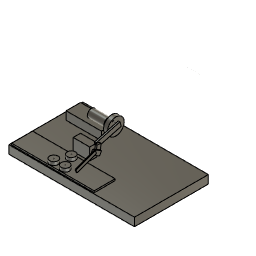
ta202 (Autodesk Fusion 360 design; units mm, degrees)
Autodesk Fusion 360 part; units mm, degrees
sketch "Sketch1" plane through (0, 0, 0) normal (0, 0, 1) x (1, 0, 0)
  line L0 (-76.1031, 44.7508) -> (76.1031, 44.7508)
  line L1 (76.1031, 44.7508) -> (76.1031, -44.7508)
  line L2 (76.1031, -44.7508) -> (-76.1031, -44.7508)
  line L3 (-76.1031, -44.7508) -> (-76.1031, 44.7508)
  line L4 (-76.1031, 44.7508) -> (76.1031, -44.7508) construction
  line L5 (76.1031, 44.7508) -> (-76.1031, -44.7508) construction
  constraint horizontal L0
  constraint perpendicular L0 L1
  constraint parallel L0 L2
  constraint parallel L1 L3
  constraint coincident L4 origin
  constraint coincident L5 origin
extrude "Extrude1" add sketch "Sketch1" along normal blind 10 makes body 1
sketch "Sketch2" plane through (0, 0, 0) normal (1, 0, 0) x (0, 1, 0)
sketch "Sketch3" plane through (0, 0, 0) normal (1, 0, 0) x (0, 1, 0)
box "BoxPrimitive1" add length 17.418 width 42.875 height 10 placed x (0, 1, 0) y (-1, 0, 0) z (0, 0, 1) at (-24.1172, 15.5422, 10) bodies 1
cylinder "CylinderPrimitive1" add diameter 10 height 20 placed x (0, 0, -1) y (0, 1, 0) z (1, 0, 0) at (0, -41.073, 85.0863) separate body makes body 2
move_face "MoveFace1" to x (1, 0, 0) y (0, 1, 0) z (0, 0, 1) at (28.6144, 17.449, -15.0737) 1 faces at (13.3333, -41.5709, 80.1111) on bodies 2
move_body "Move1" bodies 2 to x (1, 0, 0) y (0, 1, 0) z (0, 0, 1) at (-43.6789, 0, -44.4828)
sketch "Sketch6" plane through (0, 0, 0) normal (0, 1, 0) x (1, 0, 0)
move_face "MoveFace2" to x (1, 0, 0) y (0, 1, 0) z (0, 0, 1) at (0.268, 46.6265, 0) 1 faces at (-30.3455, -24.1219, 20.5547) on bodies 2
sketch "Sketch7" plane through (0, 0, 0) normal (1, 0, 0) x (0, 1, 0)
cylinder "CylinderPrimitive2" add diameter 2 height 5 placed x (0, 0, -1) y (0, 1, 0) z (1, 0, 0) at (0, -168.074, 163.9836) separate body makes body 3
move_body "Move2" bodies 3 to x (1, 0, 0) y (0, 1, 0) z (0, 0, 1) at (-21.4514, 191.469, -137.4249)
move_body "Move3" bodies 3 to x (1, 0, 0) y (0, 1, 0) z (0, 0, 1) at (-2.3482, -0.1768, -0.4425)
form "Form1" [no effect]
cylinder "CylinderPrimitive3" add diameter 20 height 5 placed x (0, 0, -1) y (0, 1, 0) z (1, 0, 0) at (0, -147.6464, 105.2635) separate body makes body 4
move_body "Move4" bodies 4 to x (1, 0, 0) y (0, 1, 0) z (0, 0, 1) at (-20, 171.5411, -79.8958)
sketch "Sketch10" plane through (0, 0, 0) normal (1, 0, 0) x (0, 1, 0)
  line L0 (-210, 70) -> (-180, 70)
  line L1 (-180, 70) -> (-180, 75.6661)
  line L2 (-180, 75.6661) -> (-210, 75.6661)
  line L3 (-210, 75.6661) -> (-210, 70)
  dimension "d14" = 30
  constraint horizontal L0
  constraint vertical L1
  constraint horizontal L2
  constraint vertical L3
  measures "d14" distance of L0.start L0.end
extrude "Extrude2" add sketch "Sketch10" along normal blind 2 separate body makes body 5
cylinder "CylinderPrimitive4" add diameter 2 height 5 placed x (0, 0, -1) y (0, 1, 0) z (1, 0, 0) at (0, -197.7484, 45.2843) separate body makes body 6
move_body "Move5" bodies 6 to x (1, 0, 0) y (0, 1, 0) z (0, 0, 1) at (-15.3609, 222.8611, -18.3783)
move_face "MoveFace3" by (0, -1.6884, -1.1256) 1 faces at (-10.3609, 25.332, 26.6123) on bodies 6
move_face "MoveFace4" to x (1, 0, 0) y (0, 1, 0) z (0, 0, 1) at (0, 0.149, -0.9888) 1 faces at (-13.6943, 25.7165, 26.1088) on bodies 6
move_body "Move6" bodies 6 to x (1, 0, 0) y (0, 1, 0) z (0, 0, 1) at (0, -2, 0)
move_body "Move7" bodies 5 to x (1, 0, 0) y (0, 1, 0) z (0, 0, 1) at (-10, 204.5024, -47.2747)
box "BoxPrimitive2" cut length 14.5484 width 8.8654 height 20 placed x (0, 0, -1) y (0, 1, 0) z (1, 0, 0) at (0, -5.9103, 24.2811) bodies 1
extrude "Extrude3" add 1 faces at (6.6667, -2.9551, 9.7327) along direction (0, 0, 1) blind 12 on bodies 1 bodies 1
move_face "MoveFace5" by (-30, 0, 3) 5 faces at (6.6667, -5.9103, 13.9109) (6.6667, -2.9551, 21.7327) (20, -2.9551, 13.9109) (6.6667, 2.9551, 13.9109) (0, -2.9551, 13.9109) on bodies 1
move_face "MoveFace6" by (0, -7, 0) 5 faces at (-10, -2.9551, 14.9109) (-23.3333, -2.9551, 24.7327) (-30, -2.9551, 14.9109) (-16.6667, 2.9551, 19.8218) (-23.3333, -5.9103, 14.9109) on bodies 1
sketch "Sketch13" plane through (0, 0, 0) normal (1, 0, 0) x (0, 1, 0)
  line L0 (-120, 50) -> (-115, 50)
  line L1 (-115, 50) -> (-115, 40)
  line L2 (-115, 40) -> (-120, 40)
  line L3 (-120, 40) -> (-120, 50)
  dimension "d26" = 5
  constraint horizontal L0
  constraint vertical L1
  constraint horizontal L2
  constraint vertical L3
  measures "d26" distance of L0.start L0.end
extrude "Extrude4" add sketch "Sketch13" along normal blind 2 separate body makes body 7
move_body "Move8" bodies 7 to x (1, 0, 0) y (0, 0.939693, -0.34202) z (0, 0.34202, 0.939693) at (-8, 89.0673, -60.0772)
sketch "Sketch14" plane through (0, 0, 0) normal (1, 0, 0) x (0, 1, 0)
  line L0 (-145, 55) -> (-140, 55)
  line L1 (-140, 55) -> (-140, 45)
  line L2 (-140, 45) -> (-145, 45)
  line L3 (-145, 45) -> (-145, 55)
  dimension "d29" = 5
  constraint horizontal L0
  constraint vertical L1
  constraint horizontal L2
  constraint vertical L3
  measures "d29" distance of L0.start L0.end
extrude "Extrude5" add sketch "Sketch14" along normal blind 2 separate body makes body 8
move_body "Move9" bodies 8 to x (1, 0, 0) y (0, 0.5, 0.866025) z (0, -0.866025, 0.5) at (7, 104.478, 118.4178)
move_body "Move10" bodies 8 to x (1, 0, 0) y (0, 1, 0) z (0, 0, 1) at (-12, 0, 0)
move_body "Move11" bodies 8 to x (1, 0, 0) y (0, 1, 0) z (0, 0, 1) at (-1, 0, 0)
sketch "Sketch15" plane through (0, 0, 0) normal (0, 0, 1) x (1, 0, 0)
  line L0 (-76.9244, -18.2082, -18.2082) -> (23.0756, -18.2082, -18.2082)
  line L1 (23.0756, -18.2082, -18.2082) -> (23.0756, -43.5769, -18.2082)
  line L2 (23.0756, -43.5769, -18.2082) -> (-76.9244, -43.5769, -18.2082)
  line L3 (-76.9244, -43.5769, -18.2082) -> (-76.9244, -18.2082, -18.2082)
  dimension "d32" = 100
extrude "Extrude6" add sketch "Sketch15" along normal blind 2 separate body contours L0 L1 L2 L3 in plane through (0, 0, -18.2082) normal (0, 0, 1) makes body 9
move_body "Move12" bodies 9 to x (1, 0, 0) y (0, 1, 0) z (0, 0, 1) at (2, 0, 30)
move_body "Move13" bodies 9 to x (1, 0, 0) y (0, 1, 0) z (0, 0, 1) at (0, 0, -1.5)
move_body "Move14" bodies 9 to x (1, 0, 0) y (0, 1, 0) z (0, 0, 1) at (1.0229, 0, -0.2046)
move_body "Move15" bodies 6 3 5 7 to x (1, 0, 0) y (0, 0.965926, 0.258819) z (0, -0.258819, 0.965926) at (0, 5.4495, 1.0154)
cylinder "CylinderPrimitive5" add diameter 10 height 4 placed x (1, 0, 0) y (0, 1, 0) z (0, 0, 1) at (-90, -90, 10) separate body makes body 10
cylinder "CylinderPrimitive6" add diameter 10 height 4 placed x (1, 0, 0) y (0, 1, 0) z (0, 0, 1) at (-72.4232, -90.9123, 10) separate body makes body 11
cylinder "CylinderPrimitive7" add diameter 10 height 4 placed x (1, 0, 0) y (0, 1, 0) z (0, 0, 1) at (-55, -90, 10) separate body makes body 12
move_body "Move16" bodies 12 to x (1, 0, 0) y (0, 1, 0) z (0, 0, 1) at (33.8754, 66.998, 2.0702)
move_body "Move17" bodies 11 to x (1, 0, 0) y (0, 1, 0) z (0, 0, 1) at (57.7763, 53.0714, 2)
move_body "Move18" bodies 10 to x (1, 0, 0) y (0, 1, 0) z (0, 0, 1) at (61.5403, 52.1304, 2)
move_face "MoveFace7" to x (1, 0, 0) y (0, 1, 0) z (0, 0, 1) at (-1, 0, 0) 2 faces at (-19.3173, -21.0864, 16.0702) (-16.1495, -23.4999, 14.7368) on bodies 12
sketch "Sketch21" plane through (0, 0, 0) normal (1, 0, 0) x (0, 1, 0)
sketch "Sketch22" plane through (0, 0, 0) normal (0, 0, 1) x (1, 0, 0)
cylinder "CylinderPrimitive8" add diameter 0.02 height 25 placed x (0, 0, -1) y (0, 1, 0) z (1, 0, 0) at (0, 91.7998, 62.8457) separate body makes body 13
cylinder "CylinderPrimitive11" add diameter 1 height 1 placed x (0, 0, -1) y (0, 1, 0) z (1, 0, 0) at (0, 68.333, 32.3551) separate body makes body 14
cylinder "CylinderPrimitive12" add diameter 1 height 1 placed x (0, 0, -1) y (0, 1, 0) z (1, 0, 0) at (0, 70, 25) separate body makes body 15
cylinder "CylinderPrimitive13" add diameter 1 height 1 placed x (0, 0, -1) y (0, 1, 0) z (1, 0, 0) at (0, 78.651, 31.8595) separate body makes body 16
cylinder "CylinderPrimitive14" add diameter 1 height 1 placed x (0, 0, -1) y (0, 1, 0) z (1, 0, 0) at (0, 78.067, 24.0747) separate body makes body 17
move_body "Move19" bodies 17 to x (1, 0, 0) y (0, 1, 0) z (0, 0, 1) at (-5.629, -57.3883, 8.9477)
move_body "Move20" bodies 15 to x (1, 0, 0) y (0, 1, 0) z (0, 0, 1) at (-1.28, -77.2263, -5.113)
move_body "Move21" bodies 14 to x (1, 0, 0) y (0, 1, 0) z (0, 0, 1) at (-1.0781, -73.9254, -5.2956)
box "BoxPrimitive4" add length 25 width 4 height 1 placed x (0, 0, 1) y (1, 0, 0) z (0, 1, 0) at (-140, 0, -79.9465) separate body makes body 18
move_body "Move23" bodies 18 to x (0, 0.173648, -0.984808) y (-1, 0, 0) z (0, 0.984808, 0.173648) at (-6.9176, 53.861, -89.1067)
move_body "Move24" bodies 18 to x (1, 0, 0) y (0, 0.984808, 0.173648) z (0, -0.173648, 0.984808) at (0, 5.6503, 6.4545)
move_body "Move25" bodies 18 to x (1, 0, 0) y (0, 1, 0) z (0, 0, 1) at (0, 12.2319, -16.2718)
move_body "Move26" bodies 14 to x (1, 0, 0) y (0, 1, 0) z (0, 0, 1) at (-5, 0, -2)
move_body "Move27" bodies 15 to x (1, 0, 0) y (0, 1, 0) z (0, 0, 1) at (-2, 0, -1)
move_body "Move28" bodies 15 to x (1, 0, 0) y (0, 1, 0) z (0, 0, 1) at (-1, 0, 0)
move_body "Move29" bodies 8 18 to x (1, 0, 0) y (0, 1, 0) z (0, 0, 1) at (20, 0, 0)
move_body "Move30" bodies 8 to x (1, 0, 0) y (0, 1, 0) z (0, 0, 1) at (-20, 0, 0)
move_body "Move31" bodies 18 to x (1, 0, 0) y (0, 1, 0) z (0, 0, 1) at (-16, 0, 0)
move_body "Move32" bodies 16 to x (1, 0, 0) y (0, 1, 0) z (0, 0, 1) at (-2.5, -92.2069, -9.2778)
move_body "Move33" bodies 16 to x (1, 0, 0) y (0, 1, 0) z (0, 0, 1) at (-0.3, 0, 0)
hole "Hole1" at (-28.4597, -37.8696, 16) direction (0, 0, -1) diameter 0.5 depth 0.5 tip angle 118 bodies 10
move_face "MoveFace10" to x (1, 0, 0) y (0, 1, 0) z (0, 0, 1) at (-9, 0, 0) 1 faces at (-5.2957, 20.873, 32.5616) on bodies 17
move_body "Move34" bodies 17 to x (1, 0, 0) y (0, 1, 0) z (0, 0, 1) at (-3, 0, 0)
move_body "Move35" bodies 3 to x (1, 0, 0) y (0, 1, 0) z (0, 0, 1) at (-0.4372, 12.8428, -5.7212)
move_body "Move36" bodies 3 to x (1, 0, 0) y (0, 1, 0) z (0, 0, 1) at (0, -11.1491, -0.6558)
hole "Hole2" at (-14.6468, -37.8409, 16) direction (0, 0, -1) diameter 0.5 depth 10 tip angle 118 bodies 1 9 11
hole "Hole3" at (-22.0108, -22.8882, 16.0702) direction (0, 0, -1) diameter 0.5 depth 10 tip angle 118 bodies 1 9 12
